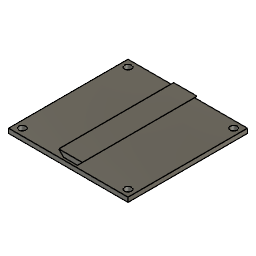
base_bottom (Autodesk Fusion 360 design; units mm, degrees)
part number: 2026-03-16-14-32-38-053
Autodesk Fusion 360 part; units mm, degrees
sketch "Sketch5" plane through (0, 0, 0) normal (0, 0, 1) x (1, 0, 0)
  line L0 (66.04, -66.04) -> (-66.04, -66.04)
  line L1 (-66.04, -66.04) -> (-66.04, 66.04)
  line L2 (-66.04, 66.04) -> (66.04, 66.04)
  line L3 (66.04, 66.04) -> (66.04, -66.04)
  line L4 (66.04, -66.04) -> (-66.04, 66.04) construction
  line L5 (-66.04, -66.04) -> (66.04, 66.04) construction
  constraint horizontal L0
  constraint perpendicular L0 L1
  constraint parallel L0 L2
  constraint parallel L1 L3
  constraint coincident L4 origin
  constraint coincident L5 origin
extrude "Extrude8" add sketch "Sketch5" along normal blind 5.08 makes body 1
sketch "Sketch6" plane through (0, 0, 5.08) normal (0, 0, 1) x (-1, 0, 0)
  line L0 (-66.04, -66.04) -> (66.04, -66.04)
  line L1 (66.04, -66.04) -> (66.04, 66.04)
  line L2 (66.04, 66.04) -> (-66.04, 66.04)
  line L3 (-66.04, 66.04) -> (-66.04, -66.04)
  circle A0 centre (58.42, -58.42) radius 3.81
  circle A1 centre (-58.42, -58.42) radius 3.81
  circle A2 centre (58.42, 58.42) radius 3.81
  circle A3 centre (-58.42, 58.42) radius 3.81
  dimension "d26" = 7.62
  dimension "d27" = 7.62
  dimension "d28" = 7.62
  dimension "d29" = 7.62
  measures "d26" diameter of A0
  measures "d27" diameter of A1
  measures "d28" diameter of A2
  measures "d29" diameter of A3
extrude "Extrude9" cut sketch "Sketch6" against normal blind 15.24 contours A0 | A1 | A2 | A3 bodies 1
sketch "Sketch7" plane through (0, 0, 5.08) normal (0, 0, 1) x (-1, 0, 0)
  circle A0 centre (58.42, -58.42) radius 3.81
  circle A1 centre (-58.42, -58.42) radius 3.81
  circle A2 centre (58.42, 58.42) radius 3.81
  circle A3 centre (-58.42, 58.42) radius 3.81
  line L0 (-66.04, -66.04) -> (66.04, -66.04)
  line L1 (66.04, -66.04) -> (66.04, 66.04)
  line L2 (66.04, 66.04) -> (-66.04, 66.04)
  line L3 (-66.04, 66.04) -> (-66.04, -66.04)
  circle A4 centre (0, 0) radius 62.8904
  dimension "d32" = 125.7808
  constraint coincident A4.centre origin
  measures "d32" diameter of A4
sketch "Sketch8" plane through (0, 0, 0) normal (0, 1, 0) x (1, 0, 0)
  line L0 (-7.62, -7.62) -> (-13.006, -13.0103)
  line L1 (7.62, -7.62) -> (13.0103, -13.006)
  line L2 (13.0103, -13.006) -> (-13.006, -13.0103)
  line L3 (7.62, -7.62) -> (-7.62, -7.62)
  dimension "d35" = 7.62
  dimension "d36" = 7.62
  constraint perpendicular L0 L1
  constraint horizontal L3
  measures "d35" distance of L0.start L0.end
  measures "d36" distance of L1.start L1.end
extrude "Extrude11" add sketch "Sketch8" along normal blind 63.5 and the other way blind 63.5 separate body makes body 2
move_body "Move1" bodies 2 to x (1, 0, 0) y (0, 1, 0) z (0, 0, 1) at (-0.0004, 0, -2.54)
